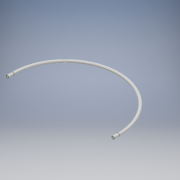
# Autodesk Inventor part: Петля
Saved by Autodesk Inventor 2017 (Build 210142000, 142)
## iProperties
Part Number: Петля
Material: Типовые
Document SubType Name: Modeling
Designer: Daemon
Density: 1 g/cm^3
Appearance: По умолчанию
Author: Daemon
Autodesk Inventor part; units mm, degrees
ref_plane "YZ Plane" through (0, 0, 0) normal (1, 0, 0) x (0, 1, 0)
ref_plane "XZ Plane" through (0, 0, 0) normal (0, 1, 0) x (-1, 0, 0)
ref_plane "XY Plane" through (0, 0, 0) normal (0, 0, 1) x (1, 0, 0)
sketch "Эскиз1" plane through (0, 0, 0) normal (0, 0, 1) x (1, 0, 0)
  arc A0 (40, 2) -> (0, 2) centre (20, 2) ccw
  line L0 (0, 0) -> (0, 2)
  line L1 (40, 0) -> (40, 2)
  point P0 (0, 0)
  point P1 (20, 22)
  dimension "d4" = 40
  dimension "d15" = 22
  constraints: 4 end point, 3 point on circle, 2 tangent, 2 vertical, 1 centre point, 1 coincident, 1 parallel
  measures "d4" distance between parallel lines of L0 L1
  measures "d15" vertical distance of L1.start point (20, 22)
sketch "Эскиз3" plane through (0, 0, 0) normal (0, 1, 0) x (-1, 0, 0)
  circle A0 centre (0, 0) radius 0.5
  dimension "d11" = 1
  constraints: 1 centre point, 1 coincident
  measures "d11" diameter of A0
sweep "Сдвиг1" add profiles "Эскиз3" path "Эскиз1"
